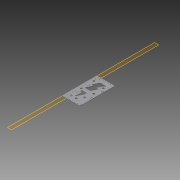
# Autodesk Inventor part: talon plate
Saved by Autodesk Inventor 2015 (Build 190159000, 159)
## iProperties
Created: 2015-02-10
Part Number: talon plate
Material: Generic
Document SubType Name: Modeling
Designer: sspriggs
Density: 1 g/cm^3
Appearance: Default
Mass: 29.8434 g
Surface Area: 293.81 cm^2
Volume: 29.8434 cm^3
Author: sspriggs
Autodesk Inventor part; units mm, degrees
ref_plane "YZ Plane" through (0, 0, 0) normal (1, 0, 0) x (0, 1, 0)
ref_plane "XZ Plane" through (0, 0, 0) normal (0, 1, 0) x (-1, 0, 0)
ref_plane "XY Plane" through (0, 0, 0) normal (0, 0, 1) x (1, 0, 0)
ref_plane "Work Plane1" through (-2.7575, 14.1676, 33.7809) normal (0, 1, 0) x (1, 0, 0)
sketch "Sketch1" plane through (-2.7575, 14.1676, 33.7809) normal (0, 1, 0) x (1, 0, 0)
  line L0 (-6.2522, 80.2164) -> (82.6478, 80.2164)
  line L1 (82.6478, 80.2164) -> (82.6478, -97.5836)
  line L2 (82.6478, -97.5836) -> (-6.2522, -97.5836)
  line L3 (-6.2522, -97.5836) -> (-6.2522, 80.2164)
  point P0 (2.7575, 33.7809)
  dimension "d0" = 177.8
  dimension "d1" = 88.9
  constraints: 8 end point, 2 parallel, 1 horizontal, 1 perpendicular
  measures "d0" distance of L0.end L1.end
  measures "d1" distance of L1.end L2.end
extrude "Extrusion1" add sketch "Sketch1" along normal blind 2.286
sketch "Sketch2" plane through (-2.7575, 16.4536, 33.7809) normal (0, 1, 0) x (1, 0, 0)
  line L0 (82.6478, 80.2164) -> (-6.2522, 80.2164) projected
  line L1 (-6.2522, 80.2164) -> (-6.2522, -97.5836) projected
  line L2 (-6.2522, -97.5836) -> (82.6478, -97.5836) projected
  line L3 (82.6478, -97.5836) -> (82.6478, 80.2164) projected
  circle A0 centre (5.0092, 73.556) radius 1.6383
  circle A1 centre (5.0092, 60.856) radius 1.6383
  circle A2 centre (5.0092, -2.644) radius 1.6383
  circle A3 centre (5.0092, -78.844) radius 1.6383
  circle A4 centre (5.0092, -91.544) radius 1.6383
  circle A5 centre (5.0092, -40.744) radius 1.6383
  circle A6 centre (5.0092, -53.444) radius 1.6383
  circle A7 centre (5.0092, 10.056) radius 1.6383
  constraints: 8 centre point
extrude "Extrusion2" cut sketch "Sketch2" against normal blind 2.286 contours A0 | A1 | A2 | A3 | A4 | A5 | A6 | A7
sketch "Sketch3" plane through (-2.7575, 16.4536, 33.7809) normal (0, 1, 0) x (1, 0, 0)
  line L0 (82.6478, -97.5836) -> (-6.2522, -97.5836) projected
  line L1 (82.6478, 80.2164) -> (-6.2522, 80.2164) projected
  point P0 (2.7575, 33.7809)
  point P1 (17.1634, 76.4064)
  point P2 (17.1634, -93.7736)
  dimension "d7" = 3.81
  dimension "d8" = 3.81
  constraints: 1 vertical alignment
  measures "d7" distance from line of L0 point (17.163, -93.774)
  measures "d8" distance from line of L1 point (17.163, 76.406)
hole "Hole1" at (14.406, 16.4536, -42.6255) at (14.406, 16.4536, 127.5545) direction (0, -1, 0) diameter 3.2766 depth 2.286 tip angle 118
pattern_linear "Rectangular Pattern1" count 5 spacing 12.7 along (1, 0, 0) of "Hole1"
sketch "Sketch4" plane through (-2.7575, 14.1676, 33.7809) normal (0, -1, 0) x (1, 0, 0)
  circle A0 centre (17.0306, -68.4388) radius 2.1989
  circle A1 centre (79.159, -26.6304) radius 2.1723
  circle A2 centre (79.159, 30.2438) radius 2.1723
  circle A3 centre (17.0306, -11.5646) radius 1.945
  circle A4 centre (79.159, 87.0884) radius 1.9184
  circle A5 centre (17.0306, 45.28) radius 2.1989
  circle A6 centre (17.0306, -19.6986) radius 1.945
  circle A7 centre (17.0306, 37.6648) radius 1.945
  circle A8 centre (79.159, -19.6986) radius 2.1723
  circle A9 centre (79.159, 37.6648) radius 2.1723
  point P0 (2.7575, -33.7809)
  constraints: 10 centre point, 4 equal radius
extrude "Extrusion3" cut sketch "Sketch4" against normal blind 2.286
sketch "Sketch6" plane through (79.8904, 14.1676, 131.3645) normal (1, 0, 0) x (0, 0, -1)
  line L0 (177.8, 2.286) -> (0, 2.286)
  line L1 (0, 2.286) -> (0, 0)
  line L2 (0, 0) -> (177.8, 0)
  line L3 (177.8, 0) -> (177.8, 2.286)
  point P0 (131.3645, -14.1676)
  constraints: 8 end point, 2 parallel, 1 horizontal, 1 perpendicular
extrude "Extrusion4" add sketch "Sketch6" along normal blind 2.286
fillet "Fillet2" radius 6.35 2 edges at (82.1764, 15.3106, 131.3645) (82.1764, 15.3106, -46.4355)
sketch "Sketch7" plane through (-2.7575, 16.4536, 33.7809) normal (0, 1, 0) x (1, 0, 0)
  line L0 (34.7695, 56.861) -> (65.3604, 56.861)
  line L1 (65.3604, 56.861) -> (45.2663, 24.4707)
  line L2 (45.2663, 24.4707) -> (59.3621, 24.4707)
  line L3 (59.3621, 24.4707) -> (45.2663, -4.6207)
  line L4 (45.2663, -4.6207) -> (55.3134, -4.6207)
  line L5 (55.3134, -4.6207) -> (42.7117, -30.6284)
  line L6 (42.7117, -30.6284) -> (47.3657, -30.6284)
  line L7 (47.3657, -30.6284) -> (34.7695, -57.0213)
  line L8 (34.7695, 56.861) -> (19.6872, 25.7339)
  line L9 (19.6872, 25.7339) -> (30.5707, 25.7339)
  line L10 (30.5707, 25.7339) -> (16.34, -4.6207)
  line L11 (16.34, -4.6207) -> (27.2284, -4.6207)
  line L12 (27.2284, -4.6207) -> (19.6872, -30.6284)
  line L13 (19.6872, -30.6284) -> (30.5707, -30.6284)
  line L14 (30.5707, -30.6284) -> (27.2284, -67.2133)
  line L15 (27.2284, -67.2133) -> (34.7695, -57.0213)
  point P0 (2.7575, 33.7809)
  constraints: 32 end point, 4 horizontal, 4 parallel
extrude "Extrusion5" cut sketch "Sketch7" against normal blind 25.4
sketch "Sketch8" plane through (-2.7575, 16.4536, 33.7809) normal (0, 1, 0) x (1, 0, 0)
  circle A0 centre (11.4041, 48.0023) radius 5.08
  circle A1 centre (66.6972, 39.8108) radius 5.08
  circle A2 centre (66.6972, -8.8344) radius 5.08
  circle A3 centre (58.9374, -47.6638) radius 5.08
  circle A4 centre (42.4705, -73.279) radius 5.08
  circle A5 centre (16.4841, -73.279) radius 5.08
  circle A6 centre (11.4041, -16.4464) radius 5.08
  point P0 (2.7575, 33.7809)
  dimension "d27" = 10.16
  dimension "d28" = 10.16
  dimension "d29" = 10.16
  dimension "d30" = 10.16
  dimension "d31" = 10.16
  dimension "d32" = 10.16
  dimension "d33" = 10.16
  constraints: 7 centre point
  measures "d27" diameter of A0
  measures "d28" diameter of A1
  measures "d29" diameter of A2
  measures "d30" diameter of A3
  measures "d31" diameter of A4
  measures "d32" diameter of A5
  measures "d33" diameter of A6
extrude "Extrusion6" cut sketch "Sketch8" against normal blind 25.4
sketch "Sketch9" plane through (-2.7575, 16.4536, 33.7809) normal (0, 1, 0) x (1, 0, 0)
  line L0 (19.6872, -30.6284) -> (27.2284, -4.6207) projected
  line L1 (21.9778, -22.7287) -> (55.3134, -22.7287)
  line L2 (55.3134, -22.7287) -> (55.3134, -4.6207)
  line L3 (55.3134, -4.6207) -> (21.9778, -4.6207)
  line L4 (21.9778, -4.6207) -> (21.9778, -22.7287)
  point P0 (2.7575, 33.7809)
  constraints: 8 end point, 2 parallel, 1 horizontal, 1 perpendicular, 1 point on line
extrude "Extrusion7" add sketch "Sketch9" against normal blind 2.286
equation "\"d8\" = d7"
body "Solid1"
